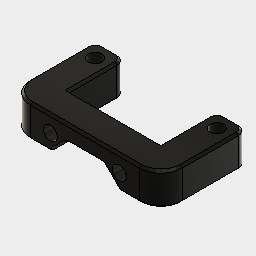
Encoder Mount (Autodesk Fusion 360 design; units mm, degrees)
Autodesk Fusion 360 part; units mm, degrees
note: some values were not read from the file. Set by a fixed rule: which sketch regions a step uses.
sketch "Sketch1" plane through (0, 0, 0) normal (0, 1, 0) x (1, 0, 0)
  circle A0 centre (-14.1, 0) radius 1.6
  circle A1 centre (14.1, 0) radius 1.6
  line L0 (17.6, 1.5) -> (17.6, -11.5)
  line L1 (12.6, -16.5) -> (-12.6, -16.5)
  line L2 (-17.6, -11.5) -> (-17.6, 1.5)
  line L3 (10.6, 1.5) -> (10.6, -7.5)
  line L4 (-10.6, -7.5) -> (-10.6, 1.5)
  line L5 (12.6, 3.5) -> (15.6, 3.5)
  line L6 (-15.6, 3.5) -> (-12.6, 3.5)
  arc A2 (-17.6, -11.5) -> (-12.6, -16.5) centre (-12.6, -11.5) ccw
  arc A3 (12.6, -16.5) -> (17.6, -11.5) centre (12.6, -11.5) ccw
  arc A4 (-15.6, 3.5) -> (-17.6, 1.5) centre (-15.6, 1.5) ccw
  arc A5 (-10.6, 1.5) -> (-12.6, 3.5) centre (-12.6, 1.5) ccw
  arc A6 (12.6, 3.5) -> (10.6, 1.5) centre (12.6, 1.5) ccw
  arc A7 (17.6, 1.5) -> (15.6, 3.5) centre (15.6, 1.5) ccw
  line L7 (10.6, -7.5) -> (10.6, -9.5)
  line L8 (10.6, -9.5) -> (-10.6, -9.5)
  line L9 (-10.6, -9.5) -> (-10.6, -7.5)
  dimension "d2" = 14.1
  dimension "d3" = 3.2
  dimension "d4" = 3.2
  dimension "d11" = 5
  dimension "d12" = 2
  measures "d2" distance of origin A0.centre
  measures "d3" diameter of A0
  measures "d4" diameter of A1
  measures "d11" radius of A2
  measures "d12" radius of A4
extrude "Extrude1" add sketch "Sketch1" along normal blind 7.5
sketch "Sketch2" plane through (0, 0, 9.5) normal (0, 0, -1) x (1, 0, 0)
  line L0 (8.6, 0) -> (-8.6, 0)
  line L1 (-12.6, 0) -> (12.6, 0)
  line L2 (-8, 0) -> (-2.6967, 0) construction
  line L3 (-12.6, 0) -> (12.6, 0)
  line L4 (10.6, 0) -> (-10.6, 0)
  line L5 (-10.6, 0) -> (-10.6, -7.5)
  line L6 (-10.6, -7.5) -> (10.6, -7.5)
  line L7 (10.6, -7.5) -> (10.6, 0)
  circle A0 centre (8, -3.75) radius 1.6
  line L8 (-12.6, -7.5) -> (-12.6, 0)
  line L9 (8, 0) -> (4.25, -3.75)
  line L10 (12.6, -7.5) -> (-12.6, -7.5)
  line L11 (0, -3.75) -> (8, -3.75)
  circle A1 centre (-8, -3.75) radius 1.6
  line L12 (12.6, 0) -> (12.6, -7.5)
  line L13 (-8, 0) -> (-4.25, -3.75)
  line L14 (0, -3.75) -> (-8, -3.75)
  point P0 (0, -3.75)
extrude "Extrude2" cut sketch "Sketch2" against normal blind 8 contours L0 L1 L3 L4 L9 L11 L13 L14 | A0 | A1
fillet "Fillet2" radius 1 4 edges at (-8, 0, 13) (-4.25, 3.75, 13) (4.25, 3.75, 13) (8, 0, 13)
chamfer "Chamfer5" distance 0.5 angle 45 44 edges at (-10.6, 7.5, 4) (-11.1858, 7.5, -2.9142) (-14.1, 7.5, -3.5) (-17.0142, 7.5, -2.9142) (-17.6, 7.5, 5) (-16.1355, 7.5, 15.0355) (0, 7.5, 16.5) (16.1355, 7.5, 15.0355) (17.6, 7.5, 5) (17.0142, 7.5, -2.9142) (14.1, 7.5, -3.5) (11.1858, 7.5, -2.9142) (10.6, 7.5, 4) (0, 7.5, 9.5) (-10.6, 0, 4) (-11.1858, 0, -2.9142) (-14.1, 0, -3.5) (-17.0142, 0, -2.9142) (-17.6, 0, 5) (-16.1355, 0, 15.0355) (-10.5071, 0, 16.5) (-8.0315, 0.0761, 16.5) (-6.125, 1.875, 16.5) (-4.2185, 3.6739, 16.5) (0, 3.75, 16.5) (4.2185, 3.6739, 16.5) (6.125, 1.875, 16.5) (8.0315, 0.0761, 16.5) (10.5071, 0, 16.5) (16.1355, 0, 15.0355) (17.6, 0, 5) (17.0142, 0, -2.9142) (14.1, 0, -3.5) (11.1858, 0, -2.9142) (10.6, 0, 4) (9.5071, 0, 9.5) (8.0315, 0.0761, 9.5) (6.125, 1.875, 9.5) (4.2185, 3.6739, 9.5) (0, 3.75, 9.5) (-4.2185, 3.6739, 9.5) (-6.125, 1.875, 9.5) (-8.0315, 0.0761, 9.5) (-9.5071, 0, 9.5)
